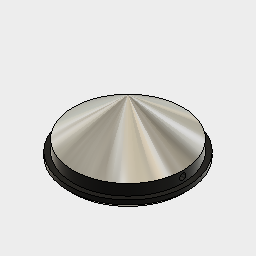
Camera Cap (Autodesk Fusion 360 design; units mm, degrees)
Autodesk Fusion 360 part; units mm, degrees
sketch "Sketch1" plane through (0, 0, 0) normal (0, 1, 0) x (1, 0, 0)
  circle A0 centre (0, 0) radius 27.5
  dimension "d1" = 55
  measures "d1" diameter of A0
extrude "Extrude1" add sketch "Sketch1" along normal blind 4
sketch "Sketch2" plane through (0, 4, 0) normal (0, 1, 0) x (-1, 0, 0)
  circle A0 centre (0, 0) radius 27.5
  circle A1 centre (0, 0) radius 25.3
  dimension "d4" = 50.6
  measures "d4" diameter of A1
extrude "Extrude2" add sketch "Sketch2" along normal blind 5 contours A1
sketch "Sketch3" plane through (0, 0, 0) normal (0, -1, 0) x (1, 0, 0)
  circle A0 centre (0, 0) radius 27.5
  line L0 (21.5985, 0) -> (19.1914, -4.1689)
  line L1 (3.5784, -14.5357) -> (-13.1761, -14.5877)
  line L2 (-11.9706, 0) -> (-14.3773, 4.1693)
  line L3 (-14.3773, 4.1693) -> (-5.9851, -10.3664)
  line L4 (14.3777, -4.1689) -> (6.0451, -18.7046)
  line L5 (5.9851, -10.3664) -> (3.5784, -14.5357)
  line L6 (-14.3773, 4.1693) -> (-6.0451, 18.705)
  line L7 (-5.9851, 18.705) -> (-14.3773, 4.1693)
  line L8 (-10.7992, -10.3664) -> (-19.2216, 4.1173)
  line L9 (-19.1914, 4.1693) -> (-10.7992, -10.3664)
  line L10 (-10.7992, -18.7046) -> (-13.2063, -14.5357)
  line L11 (-5.9851, -10.3664) -> (-10.7992, -10.3664)
  line L12 (-21.5985, 0) -> (-19.1914, 4.1693)
  line L13 (10.7992, 10.3668) -> (19.2216, -4.1169)
  line L14 (-10.7992, -10.3664) -> (5.9851, -10.3664)
  line L15 (-13.2063, -14.5357) -> (3.5784, -14.5357)
  line L16 (14.3777, -4.1689) -> (5.9851, 10.3668)
  line L17 (13.2063, 14.5357) -> (-3.578, 14.5357)
  line L18 (6.0451, -18.7046) -> (-10.7992, -18.7046)
  line L19 (11.9706, 0) -> (14.3777, -4.1689)
  line L20 (19.1914, -4.1689) -> (10.7992, 10.3668)
  line L21 (5.9851, -18.7046) -> (14.3777, -4.1689)
  line L22 (13.1765, 14.5877) -> (21.5985, 0)
  line L23 (-6.0451, 18.705) -> (10.7992, 18.705)
  line L24 (-3.578, 14.5357) -> (-11.9706, 0)
  line L25 (10.7992, 10.3668) -> (-5.9851, 10.3668)
  line L26 (10.7992, -18.7046) -> (5.9851, -18.7046)
  line L27 (19.2216, -4.1169) -> (10.7992, -18.7046)
  line L28 (10.7992, 18.705) -> (13.2063, 14.5357)
  line L29 (-11.9706, 0) -> (11.9706, 0)
  line L30 (0, 0) -> (0, 10.3668)
  line L31 (-19.2216, 4.1173) -> (-10.7992, 18.705)
  line L32 (-13.1761, -14.5877) -> (-21.5985, 0)
  line L33 (-10.7992, 18.705) -> (-5.9851, 18.705)
  line L34 (3.5784, -14.5357) -> (11.9706, 0)
  line L35 (5.9851, 10.3668) -> (10.7992, 10.3668)
  line L36 (-3.578, 14.5357) -> (13.1765, 14.5877)
  line L37 (-5.9851, 10.3668) -> (-3.578, 14.5357)
  line L38 (-13.2236, 4.171) -> (-5.4656, 17.705)
  line L39 (-5.4656, 17.705) -> (10.2219, 17.705)
  line L40 (10.2219, 17.705) -> (11.4743, 15.5357)
  line L41 (11.4743, 15.5357) -> (-4.1554, 15.5357)
  line L42 (-4.1554, 15.5357) -> (-11.9705, 2.0001)
  line L43 (-11.9705, 2.0001) -> (-13.2236, 4.171)
  line L44 (11.3766, 11.3668) -> (-4.253, 11.3668)
  line L45 (-4.253, 11.3668) -> (-2.9997, 13.5375)
  line L46 (-2.9997, 13.5375) -> (12.6002, 13.5859)
  line L47 (12.6002, 13.5859) -> (20.4438, 0)
  line L48 (20.4438, 0) -> (19.1914, -2.1689)
  line L49 (19.1914, -2.1689) -> (11.3766, 11.3668)
  line L50 (10.224, 9.3668) -> (18.0659, -4.1187)
  line L51 (18.0659, -4.1187) -> (10.2219, -17.7046)
  line L52 (10.2219, -17.7046) -> (7.7172, -17.7046)
  line L53 (7.7172, -17.7046) -> (15.5324, -4.1689)
  line L54 (15.5324, -4.1689) -> (7.7172, 9.3668)
  line L55 (7.7172, 9.3668) -> (10.224, 9.3668)
  line L56 (13.224, -4.1707) -> (5.4657, -17.7046)
  line L57 (5.4657, -17.7046) -> (-10.2219, -17.7046)
  line L58 (-10.2219, -17.7046) -> (-11.4742, -15.5357)
  line L59 (-11.4742, -15.5357) -> (4.1558, -15.5357)
  line L60 (4.1558, -15.5357) -> (11.9706, -2)
  line L61 (11.9706, -2) -> (13.224, -4.1707)
  line L62 (3, -13.5375) -> (-12.5998, -13.5859)
  line L63 (-12.5998, -13.5859) -> (-20.4438, 0)
  line L64 (-20.4438, 0) -> (-19.1914, 2.1693)
  line L65 (-19.1914, 2.1693) -> (-11.3766, -11.3664)
  line L66 (-11.3766, -11.3664) -> (4.2532, -11.3664)
  line L67 (4.2532, -11.3664) -> (3, -13.5375)
  line L68 (-10.224, -9.3664) -> (-18.0659, 4.1191)
  line L69 (-18.0659, 4.1191) -> (-10.2219, 17.705)
  line L70 (-10.2219, 17.705) -> (-7.7172, 17.705)
  line L71 (-7.7172, 17.705) -> (-15.532, 4.1693)
  line L72 (-15.532, 4.1693) -> (-7.7172, -9.3664)
  line L73 (-7.7172, -9.3664) -> (-10.224, -9.3664)
  dimension "d8" = 1
  dimension "d9" = 1
  dimension "d10" = 1
  dimension "d11" = 1
  dimension "d12" = 1
  dimension "d13" = 1
extrude "Extrude3" cut sketch "Sketch3" against normal blind 1 contours L38 L39 L40 L41 L42 L43 | L44 L45 L46 L47 L48 L49 | L50 L51 L52 L53 L54 L55 | L56 L57 L58 L59 L60 L61 | L62 L63 L64 L65 L66 L67 | L68 L69 L70 L71 L72 L73
chamfer "Chamfer1" distance 2 angle 45 1 edges at (-25.639, 0, 9.9444)
sketch "Sketch5" plane through (0, 0, 0) normal (0, 0, 1) x (1, 0, 0)
  line L0 (25.3, 9) -> (-25.3, 9)
  line L1 (25.3, 9) -> (0, 26.7153)
  line L2 (25.3, 9) -> (54.9449, 9) construction
  line L3 (0, 26.7153) -> (0, 9)
  line L4 (0, 26.7153) -> (0, 24.5)
  dimension "d19" = 145
  dimension "d37" = 30.8856
  measures "d19" angle of L1 L2
  measures "d37" distance of L0.start L1.end
revolve "Revolve1" add sketch "Sketch5" angle 360 about axis through (0, 1.75, 0) along (0, 1, 0)
ref_plane "WorkPlane3" through (25.3, 0, 0) normal (1, 0, 0) x (0, 1, 0)
sketch "Sketch8" plane through (25.3, 0, 0) normal (1, 0, 0) x (0, 0, -1)
  line L0 (0, 9) -> (0, 6.5)
  circle A0 centre (0, 6.5) radius 1.4
  point P0 (0, 9)
  dimension "d28" = 2.5
  dimension "d29" = 2.8
  measures "d28" distance of P0 L0.end
  measures "d29" diameter of A0
extrude "Extrude6" cut sketch "Sketch8" against normal blind 8
ref_plane "WorkPlane4" through (-25.3, 0, 0) normal (1, 0, 0) x (0, 1, 0)
sketch "Sketch9" plane through (-25.3, 0, 0) normal (1, 0, 0) x (0, 0, -1)
  line L0 (0, 9) -> (0, 6.5)
  circle A0 centre (0, 6.5) radius 1.4
  point P0 (0, 9)
  dimension "d33" = 2.5
  dimension "d34" = 2.8
  measures "d33" distance of P0 L0.end
  measures "d34" diameter of A0
extrude "Extrude7" cut sketch "Sketch9" along normal blind 8
